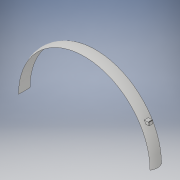
# Autodesk Inventor part: rear_light_mount
Saved by Autodesk Inventor 2019 (Build 230136000, 136)
## iProperties
Created: 2019-09-25
Part Number: rear_light_mount
Material: Generic
Document SubType Name: Modeling
Designer: Alex
Density: 1 g/cm^3
Appearance: Default
Author: Alex
Autodesk Inventor part; units mm, degrees
ref_plane "YZ Plane" through (0, 0, 0) normal (1, 0, 0) x (0, 1, 0)
ref_plane "XZ Plane" through (0, 0, 0) normal (0, 1, 0) x (-1, 0, 0)
ref_plane "XY Plane" through (0, 0, 0) normal (0, 0, 1) x (1, 0, 0)
sketch "Sketch1" plane through (0, 0, 0) normal (0, 1, 0) x (-1, 0, 0)
  line L0 (162, 9) -> (164.5, 9)
  line L1 (164.5, -10) -> (162, -10)
  line L2 (162, -10) -> (162, 9)
  line L3 (190, 11) -> (161, 11)
  line L4 (160, 10) -> (160, -11)
  line L5 (161, -12) -> (190, -12)
  line L6 (164.5, 7) -> (165.5, 7)
  line L7 (164.5, -8) -> (165.5, -8)
  line L8 (165.5, 7) -> (165.5, 5.5)
  line L9 (165.5, 5.5) -> (165.2, 5.5)
  line L10 (165.5, -8) -> (165.5, -6.5)
  line L11 (165.5, -6.5) -> (165.2, -6.5)
  line L12 (164.5, 7) -> (164.5, 9)
  line L13 (165.2, 5.5) -> (165.2, -6.5)
  line L14 (164.5, -8) -> (164.5, -10)
  arc A0 (161, 11) -> (160, 10) centre (161, 10) ccw
  arc A1 (160, -11) -> (161, -12) centre (161, -11) ccw
  line L15 (190, 11) -> (190, -12)
  point P0 (0, 0)
  dimension "d0" = 19
  dimension "d1" = 2.5
  dimension "d3" = 2
  dimension "d4" = 2
  dimension "d5" = 2
  dimension "d7" = 1
  dimension "d8" = 15
  dimension "d10" = 1.5
  dimension "d11" = 1.5
  dimension "d12" = 1
  dimension "d22" = 4
  dimension "d28" = 3.2
  dimension "d36" = 30
  dimension "d46" = 11
  dimension "d48" = 190
  constraints: 32 end point, 4 parallel, 4 point on circle, 4 tangent, 3 horizontal, 3 vertical, 2 centre point, 1 equal radius, 1 perpendicular, 1 point on line
  measures "d0" distance of L0.end L1.start
  measures "d1" distance of L1.start L1.end
  measures "d3" distance between parallel lines of L4 L2
  measures "d4" distance between parallel lines of L3 L0
  measures "d5" distance between parallel lines of L5 L1
  measures "d7" distance of L6.start L6.end
  measures "d8" distance between parallel lines of L7 L6
  measures "d10" distance of L6.end L8.end
  measures "d11" distance of L7.end L10.end
  measures "d12" radius of A0
  measures "d22" distance between parallel lines of L5 L7
  measures "d28" distance between parallel lines of L2 L13
  measures "d36" distance between parallel lines of L15 L4
  measures "d46" distance from line of point (0, 0) L3
  measures "d48" distance from line of point (0, 0) L15
extrude "Extrusion1" add sketch "Sketch1" along normal blind 16.5
sketch "Sketch5" plane through (0, 16.5, 0) normal (0, 1, 0) x (1, 0, 0)
  line L0 (-165.2, -3.25) -> (-166.2, -3.25)
  line L1 (-166.2, -3.25) -> (-166.2, 3.25)
  line L2 (-166.2, 3.25) -> (-165.2, 3.25)
  line L3 (-165.2, 3.25) -> (-165.2, -3.25)
  line L4 (-165.2, -5.5) -> (-165.2, 6.5) projected
  line L5 (-190, -11) -> (-161, -11) projected
  point P0 (0, 0)
  point P1 (-21.5, -2)
  dimension "d15" = 1
  dimension "d16" = 6.5
  dimension "d17" = 0
  dimension "d18" = 7.75
  constraints: 8 end point, 2 parallel, 1 horizontal, 1 perpendicular, 1 other
  measures "d15" distance between parallel lines of L1 L3
  measures "d16" distance between parallel lines of L2 L0
  measures "d17" distance between parallel lines of L4 L3
extrude "Extrusion2" cut sketch "Sketch5" against normal blind 15
sketch "Sketch14" plane through (0, 16.5, 0) normal (0, 1, 0) x (1, 0, 0)
  line L0 (-73.2178, -32) -> (-73.2178, 33)
  arc A0 (-73.2178, -32) -> (-73.2178, 33) centre (-121.0303, 0.5) ccw
  line L1 (-190, -11) -> (-161, -11) projected
  line L2 (-446.2178, -63.0398) -> (-446.2178, 88.5794)
  point P0 (0, 0)
  dimension "d37" = 65
  dimension "d40" = 21
  dimension "d44" = 373
  constraints: 4 end point, 2 point on circle, 2 vertical, 1 centre point
  measures "d37" distance of L0.start L0.end
  measures "d40" distance from line of L1 L0.start
  measures "d44" distance between parallel lines of L2 L0
move or copy body "Move Body2" bodies to move or copy 1 copy no translate (60, 210, 0)
revolve "Revolution1" add sketch "Sketch14" angle 180 about axis through (-446.2178, 16.5, 63.0398) along (0, 0, 1)
body "Solid1"
